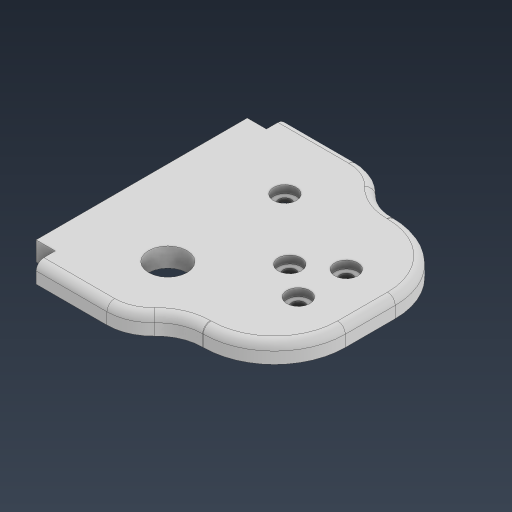
# Autodesk Inventor part: Top
Saved by Autodesk Inventor 2024 (Build 280153000, 153)
## iProperties
Created: 2023-12-19
Part Number: Top
Material: Generic
Document SubType Name: Modeling
Designer: Piter
Density: 1 g/cm^3
Appearance: Default
Author: Piter
Autodesk Inventor part; units mm, degrees
ref_plane "YZ Plane" through (0, 0, 0) normal (1, 0, 0) x (0, 1, 0)
ref_plane "XZ Plane" through (0, 0, 0) normal (0, 1, 0) x (-1, 0, 0)
ref_plane "XY Plane" through (0, 0, 0) normal (0, 0, 1) x (1, 0, 0)
sketch "Sketch1" plane through (0, 0, 0) normal (0, 1, 0) x (-1, 0, 0)
  line L0 (-25, 25) -> (25, 25)
  line L1 (25, 25) -> (25, -25)
  line L2 (25, -25) -> (-25, -25)
  line L3 (-25, -25) -> (-25, 25)
  line L4 (-25, 25) -> (25, -25) construction
  line L5 (25, 25) -> (-25, -25) construction
  line L6 (25, 0) -> (-25, 0)
  circle A0 centre (12.5, 15.25) radius 1.65
  line L7 (-25, 12.5) -> (0, 12.5)
  line L8 (-12.5, 12.5) -> (-12.5, 0)
  circle A1 centre (-12.5, 6.25) radius 1.65
  line L9 (25, -25) -> (-25, 25) construction
  circle A2 centre (12.5, -15.25) radius 1.65
  circle A3 centre (-12.5, -6.25) radius 1.65
  line L10 (0, 32.5) -> (50, 32.5)
  line L11 (50, 32.5) -> (50, -32.5)
  line L12 (50, -32.5) -> (0, -32.5)
  line L13 (0, -32.5) -> (0, 32.5)
  line L14 (0, 32.5) -> (50, -32.5) construction
  line L15 (50, 32.5) -> (0, -32.5) construction
  line L16 (50, -32.5) -> (29.5652, -32.5)
  line L17 (29.5652, -32.5) -> (29.5652, 32.5)
  line L18 (29.5652, 32.5) -> (50, 32.5)
  line L19 (0, 32.5205) -> (0, -32.5)
  circle A4 centre (12.5, -15.25) radius 15
  line L20 (29.5652, -32.5) -> (39.5652, -32.5)
  line L21 (39.5652, -32.5) -> (39.5652, 32.5)
  line L22 (39.5652, 32.5) -> (29.5652, 32.5)
  line L23 (29.5652, 32.5) -> (29.5652, -32.5)
  line L24 (12.5, -15.25) -> (12.5, 0)
  line L25 (-12.5, -6.25) -> (12.5, -6.25)
  circle A5 centre (-4, 0) radius 5
  circle A6 centre (-4, 0) radius 1.65
  line L26 (0, 0) -> (-4, 0)
  line L27 (29.5652, -32.5) -> (29.5652, -27.5)
  line L28 (29.5652, -27.5) -> (34.5652, -27.5)
  line L29 (34.5652, -27.5) -> (34.5652, 27.5)
  line L30 (34.5652, 27.5) -> (29.5652, 27.5)
  line L31 (29.5652, 27.5) -> (29.5652, -27.5)
  point P0 (0, -12.5)
  point P1 (-12.5, -12.5)
  point P2 (0, 25)
  point P3 (0, -25)
  point P4 (0, 25)
  point P5 (0, -25)
  point P6 (0, 32.5)
  point P7 (0, 32.5)
  point P8 (0, -23.5416)
  point P9 (1.101, -25)
  point P10 (25, -23.5416)
  point P11 (23.899, -25)
  point P12 (39.5652, 32.5)
  point P13 (0, 0)
  dimension "d0" = 50
  dimension "d1" = 50
  dimension "d5" = 3.3
  dimension "d7" = 3.3
  dimension "d11" = 15.25
  dimension "d12" = 50
  dimension "d13" = 65
  dimension "d19" = 30
  dimension "d21" = 10
  dimension "d27" = 7.5
  dimension "d28" = 7.5
  dimension "d31" = 9
  dimension "d32" = 25
  dimension "d57" = 10
  dimension "d58" = 3.3
  dimension "d59" = 4
  dimension "d60" = 5
  dimension "d61" = 55
  constraints: 64 end point, 10 parallel, 9 midpoint, 8 point on line, 7 centre point, 7 perpendicular, 5 horizontal, 4 symmetric about line, 2 coincident, 1 vertical, 2 other
  measures "d0" distance of L1.end L2.end
  measures "d1" distance of L0.end L1.end
  measures "d5" diameter of A0
  measures "d7" diameter of A1
  measures "d11" distance from line of A0.centre L6
  measures "d12" distance of L11.end L12.end
  measures "d13" distance of L10.end L11.end
  measures "d19" diameter of A4
  measures "d21" distance of L22.end L21.end
  measures "d27" distance between parallel lines of L2 L12
  measures "d28" distance between parallel lines of L0 L10
  measures "d31" distance from line of L25 A2.centre
  measures "d32" distance of L25.start L25.end
  measures "d57" diameter of A5
  measures "d58" diameter of A6
  measures "d59" distance of point (0, 0) L26.end
  measures "d60" distance of L16.end L27.end
  measures "d61" distance of L29.end L28.end
extrude "Extrusion3" add sketch "Sketch1" along normal blind 5 contours L0 L13 L7 L3 | L13 L10 L17 L12 L2 A4 L1 L0 | L0 L1 L6 A5 L13 | L7 L8 A1 L6 L3 | L13 A5 L6 L8 A1 L7 | L6 A5 L13 A4 L2 L3 | L1 A4 L24 L6 | A5 L6 L13 | L13 L6 A6 A5 | A4 L1 | L1 A4 L2 L13 L25 L24 | L24 A4 L25 L13 A5 L6 | L13 A5 L6 A6 | L6 A5 L13 | L30 L29 L28 L17 | L13 A4 L2 | L1 L2 A4 | L24 L25 A4 | L2 A4 | A4 L13 | A4 L13 L25 | A0
fillet "Fillet5" radius 12 2 edges at (0, 2.5, 32.5) (0, 2.5, -32.5)
fillet "Fillet6" radius 12 2 edges at (0, 2.5, 25) (0, 2.5, -25)
fillet "Fillet7" radius 18.5 2 edges at (25, 2.5, 25) (25, 2.5, -25)
sketch "Sketch5" plane through (0, 5, 0) normal (0, 1, 0) x (1, 0, 0)
  circle A0 centre (-12.5, 15.25) radius 1.65 projected
  circle A1 centre (-12.5, -15.25) radius 1.5 projected
  circle A2 centre (-12.5, -15.25) radius 5
  circle A3 centre (4, 0) radius 1.65 projected
  circle A4 centre (4, 0) radius 3
  circle A5 centre (12.5, 6.25) radius 1.65 projected
  circle A6 centre (12.5, 6.25) radius 3
  circle A7 centre (12.5, -6.25) radius 1.65 projected
  circle A8 centre (12.5, -6.25) radius 3
  circle A9 centre (-12.5, 15.25) radius 3
  point P0 (0, 0)
  dimension "d63" = 6
  dimension "d64" = 6
  dimension "d65" = 6
  dimension "d71" = 10
  dimension "d75" = 6
  constraints: 5 centre point, 5 coincident
  measures "d63" diameter of A4
  measures "d64" diameter of A6
  measures "d65" diameter of A8
  measures "d71" diameter of A2
  measures "d75" diameter of A9
extrude "Extrusion8" cut sketch "Sketch5" against normal blind 2 contours A3 | A4 | A5 | A6 | A7 | A8
fillet "Fillet9" radius 2 11 edges at (6.4021, 5, 25) (1.5607, 5, 25.9773) (-6.3809, 5, 31.5227) (-20.3448, 5, 32.5) (25, 5, 0) (19.5815, 5, -19.5815) (6.4021, 5, -25) (1.5607, 5, -25.9773) (-6.3809, 5, -31.5227) (-20.3448, 5, -32.5) (19.5815, 5, 19.5815)
extrude "Extrusion9" cut sketch "Sketch5" against normal through all contours A1 | A2
sketch "Sketch6" plane through (0, 0, 0) normal (0, -1, 0) x (1, 0, 0)
  circle A0 centre (-12.5, -15.25) radius 1.65 projected
  circle A1 centre (-12.5, -15.25) radius 5
  point P0 (0, 0)
  dimension "d72" = 10
  constraints: 1 centre point, 1 coincident
  measures "d72" diameter of A1
extrude "Extrusion10" cut sketch "Sketch6" against normal blind 2
extrude "Extrusion11" cut sketch "Sketch5" against normal blind 2 contours A0 | A9
body "Solid2"
